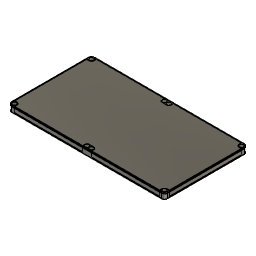
v1.0 (Autodesk Fusion 360 design; units mm, degrees)
Autodesk Fusion 360 part; units mm, degrees
sketch "Sketch1" plane through (0, 0, 0) normal (0, 0, 1) x (1, 0, 0)
  line L0 (192, -6) -> (205, -6) construction
  line L1 (192, -6) -> (179, -6) construction
  circle A0 centre (179, -188) radius 2
  circle A1 centre (13, -188) radius 2
  line L2 (13, -6) -> (13, -16) construction
  circle A2 centre (205, -16) radius 2
  line L3 (13, -198) -> (13, -188) construction
  line L4 (384, -198) -> (371, -198) construction
  line L5 (179, -26) -> (13, -26)
  line L6 (192, -198) -> (179, -198) construction
  line L7 (384, -6) -> (371, -6) construction
  line L8 (179, -6) -> (179, -26) construction
  line L9 (192, -198) -> (0, -198)
  line L10 (205, -198) -> (205, -188) construction
  line L11 (0, -198) -> (0, -6)
  circle A3 centre (179, -16) radius 2
  line L12 (384, -198) -> (384, -6)
  line L13 (371, -26) -> (205, -26)
  line L14 (371, -198) -> (371, -188) construction
  line L15 (205, -26) -> (205, -178)
  line L16 (13, -178) -> (179, -178)
  line L17 (0, -198) -> (13, -198) construction
  line L18 (205, -198) -> (205, -178) construction
  circle A4 centre (205, -188) radius 2
  line L19 (0, -198) -> (13, -198) construction
  line L20 (371, -6) -> (371, -16) construction
  line L21 (192, -6) -> (179, -6) construction
  circle A5 centre (13, -16) radius 2
  circle A6 centre (371, -16) radius 2
  line L22 (192, -6) -> (192, -198) construction
  line L23 (179, -6) -> (179, -16) construction
  line L24 (371, -6) -> (371, -26) construction
  line L25 (205, -6) -> (205, -16) construction
  line L26 (13, -26) -> (13, -178)
  line L27 (384, -6) -> (0, -6)
  line L28 (179, -198) -> (179, -188) construction
  line L29 (13, -198) -> (13, -178) construction
  line L30 (0, -6) -> (13, -6) construction
  line L31 (179, -178) -> (179, -26)
  line L32 (192, -198) -> (205, -198) construction
  line L33 (0, -6) -> (0, -198)
  line L34 (205, -178) -> (371, -178)
  circle A7 centre (371, -188) radius 2
  line L35 (384, -6) -> (371, -6) construction
  line L36 (371, -178) -> (371, -26)
  line L37 (0, -198) -> (384, -198)
  line L38 (192, -198) -> (205, -198) construction
  line L39 (384, -6) -> (384, 12) construction
  line L40 (0, -6) -> (-10.6066, 4.6066) construction
  line L41 (0, -6) -> (15, -6) construction
  circle A8 centre (-5.3033, -0.6967) radius 7.5
  line L42 (0, -198) -> (-10.6066, -208.6066) construction
  line L43 (384, -198) -> (394.6066, -208.6066) construction
  line L44 (384, -198) -> (399, -198) construction
  line L45 (384, -6) -> (394.6066, 4.6066) construction
  line L46 (384, -6) -> (399, -6) construction
  circle A9 centre (389.3033, -0.6967) radius 7.5
  circle A10 centre (389.3033, -203.3033) radius 7.5
  circle A11 centre (-5.3033, -203.3033) radius 7.5
  line L47 (-12.7709, 0) -> (-12.8033, -203.3021)
  line L48 (-5.3033, -210.8033) -> (389.3033, -210.8033)
  line L49 (396.8033, -203.3033) -> (396.8033, -0.6967)
  line L50 (-5.3033, 6.8033) -> (389.3033, 6.8033)
  point P0 (13, -13)
  dimension "d13" = 192
  dimension "d14" = 192
  dimension "d15" = 384
  dimension "d16" = 384
  dimension "d20" = 13
  dimension "d21" = 10
  dimension "d22" = 4
  dimension "d23" = 13
  dimension "d24" = 10
  dimension "d25" = 13
  dimension "d26" = 10
  dimension "d27" = 13
  dimension "d28" = 10
  dimension "d29" = 13
  dimension "d30" = 10
  dimension "d31" = 13
  dimension "d32" = 10
  dimension "d33" = 13
  dimension "d34" = 10
  dimension "d35" = 13
  dimension "d36" = 10
  dimension "d37" = 4
  dimension "d38" = 4
  dimension "d39" = 4
  dimension "d40" = 4
  dimension "d41" = 4
  dimension "d42" = 4
  dimension "d43" = 4
  dimension "d44" = 13
  dimension "d45" = 20
  dimension "d46" = 13
  dimension "d47" = 20
  dimension "d48" = 13
  dimension "d49" = 20
  dimension "d50" = 13
  dimension "d51" = 20
  dimension "d69" = 135
  dimension "d70" = 15
  dimension "d71" = 15
  dimension "d72" = 45
  dimension "d73" = 15
  dimension "d74" = 15
  dimension "d75" = 45
  constraint perpendicular L11 L30
  constraint perpendicular L2 L30
  constraint coincident L2.end A5.centre
  constraint perpendicular L7 L12
  constraint perpendicular L7 L20
  constraint perpendicular L4 L12
  constraint perpendicular L14 L37
  constraint perpendicular L19 L33
  constraint perpendicular L3 L19
  constraint midpoint L0.start L27
  constraint perpendicular L22 L37
  constraint perpendicular L6 L22
  constraint perpendicular L9 L28
  constraint perpendicular L21 L22
  constraint perpendicular L21 L23
  constraint perpendicular L0 L22
  constraint perpendicular L25 L27
  constraint perpendicular L22 L32
  constraint perpendicular L10 L32
  constraint coincident A1.centre L3.end
  constraint coincident A3.centre L23.end
  constraint coincident A0.centre L28.end
  constraint coincident A2.centre L25.end
  constraint coincident L10.end A4.centre
  constraint coincident L14.end A7.centre
  constraint coincident L20.end A6.centre
  constraint perpendicular L11 L17
  constraint perpendicular L17 L29
  constraint perpendicular L1 L22
  constraint perpendicular L1 L8
  constraint horizontal L16
  constraint vertical L31
  constraint horizontal L5
  constraint vertical L26
  constraint perpendicular L22 L38
  constraint perpendicular L18 L38
  constraint perpendicular L20 L35
  constraint perpendicular L24 L35
  constraint horizontal L34
  constraint vertical L36
  constraint horizontal L13
  constraint vertical L15
  constraint perpendicular L7 L39
  constraint horizontal L41
  constraint coincident L40.end A8
  constraint coincident L11.end A8
  constraint horizontal L44
  constraint horizontal L46
  constraint coincident L45.end A9
  constraint coincident L7.start A9
  constraint coincident L43.end A10
  constraint coincident L4.start A10
  constraint coincident L42.end A11
  constraint coincident L9.end A11
  constraint coincident A8 L47.start
  constraint coincident A11 L47.end
  constraint tangent A11 L47
  constraint coincident A11 L48.start
  constraint coincident A10 L48.end
  constraint tangent A10 L48
  constraint coincident A10 L49.start
  constraint coincident A9 L49.end
  constraint tangent A9 L49
  constraint perpendicular L46 L49
  constraint coincident A8 L50.start
  constraint coincident A9 L50.end
  constraint tangent A9 L50
  constraint perpendicular L49 L50
  measures "d13" distance of L11.end L9.end
  measures "d14" distance of L4.start L7.start
  measures "d15" distance of L7.start L11.end
  measures "d16" distance of L4.start L9.end
  measures "d20" distance of L2.start L11.end
  measures "d21" distance of L2.start L2.end
  measures "d22" diameter of A5
  measures "d23" distance of L7.end L7.start
  measures "d24" distance of L7.end L20.end
  measures "d25" distance of L4.end L4.start
  measures "d26" distance of L4.end L14.end
  measures "d27" distance of L3.start L9.end
  measures "d28" distance of L3.start A1.centre
  measures "d29" distance of L6.end L6.start
  measures "d30" distance of L6.end A0.centre
  measures "d31" distance of L0.start L1.end
  measures "d32" distance of A3.centre L1.end
  measures "d33" distance of L0.start L0.end
  measures "d34" distance of A2.centre L0.end
  measures "d35" distance of L10.start L6.start
  measures "d36" distance of L10.end L10.start
  measures "d37" diameter of A1
  measures "d38" diameter of A3
  measures "d39" diameter of A0
  measures "d40" diameter of A2
  measures "d41" diameter of A4
  measures "d42" diameter of A7
  measures "d43" diameter of A6
  measures "d44" distance of L9.end L3.start
  measures "d45" distance of L16.start L3.start
  measures "d46" distance of L0.start L1.end
  measures "d47" distance of L5.start L1.end
  measures "d48" distance of L6.start L10.start
  measures "d49" distance of L10.start L15.end
  measures "d50" distance of L7.start L7.end
  measures "d51" distance of L13.start L7.end
  measures "d69" angle of L40 L41
  measures "d70" distance of L11.end L40.end
  measures "d71" distance of L9.end L42.end
  measures "d72" angle of L43 L44
  measures "d73" distance of L4.start L43.end
  measures "d74" distance of L7.start L45.end
  measures "d75" angle of L45 L46
extrude "Extrude1" add sketch "Sketch1" along normal blind 2 contours L9 L37 A10 A11 L48 | L9 L11 L12 L27 L33 L37 | L11 L33 A8 A11 L47 | A11 | L12 A9 A10 L49 | A10 | L27 A8 A9 L50 | A8 L47 | A9 picked at (-7.7336, 1.0063) makes body 1
sketch "Sketch3" plane through (0, 0, 2) normal (0, 0, 1) x (-1, 0, 0)
  circle A0 centre (-179, 16) radius 2
  circle A1 centre (-205, 188) radius 2
  circle A2 centre (-179, 188) radius 2
  circle A3 centre (-13, 16) radius 2
  circle A4 centre (-205, 16) radius 2
  circle A5 centre (-13, 188) radius 2
  circle A6 centre (-371, 16) radius 2
  line L0 (-179, 26) -> (-179, 178)
  line L1 (-179, 178) -> (-13, 178)
  line L2 (-13, 178) -> (-13, 26)
  line L3 (-13, 26) -> (-179, 26)
  line L4 (-371, 26) -> (-371, 178)
  line L5 (-371, 178) -> (-205, 178)
  line L6 (-205, 178) -> (-205, 26)
  line L7 (-205, 26) -> (-371, 26)
  circle A7 centre (-371, 188) radius 2
  line L8 (12.7709, 0) -> (12.8033, 203.3021)
  arc A8 (12.8033, 203.3021) -> (5.3033, 210.8033) centre (5.3033, 203.3033) ccw
  line L9 (5.3033, 210.8033) -> (-389.3033, 210.8033)
  arc A9 (-389.3033, 210.8033) -> (-396.8033, 203.3033) centre (-389.3033, 203.3033) ccw
  line L10 (-396.8033, 203.3033) -> (-396.8033, 0.6967)
  arc A10 (-396.8033, 0.6967) -> (-389.3033, -6.8033) centre (-389.3033, 0.6967) ccw
  line L11 (-389.3033, -6.8033) -> (5.3033, -6.8033)
  arc A11 (5.3033, -6.8033) -> (12.7709, 0) centre (5.3033, 0.6967) ccw
  circle A12 centre (5.3033, 0.6967) radius 6.5
  circle A13 centre (5.3033, 203.3033) radius 6.5
  circle A14 centre (-389.3033, 203.3033) radius 6.5
  circle A15 centre (-389.3033, 0.6967) radius 6.5
  line L12 (-389.3033, -5.8033) -> (5.3033, -5.8033)
  line L13 (11.8033, 0.6967) -> (11.8033, 203.3033)
  line L14 (5.3033, 209.8033) -> (-389.3033, 209.8033)
  line L15 (-395.8033, 203.3033) -> (-395.8033, 0.6967)
  line L16 (-192, -5.8033) -> (-192, 209.8033) construction
  circle A16 centre (-186, 0.1967) radius 6
  circle A17 centre (-198, 0.1967) radius 6
  circle A18 centre (-186, 203.8033) radius 6
  circle A19 centre (-198, 203.8033) radius 6
  line L17 (-180, 203.8033) -> (-180, 209.8033)
  line L18 (-186, 197.8033) -> (-198, 197.8033)
  line L19 (-204, 203.8033) -> (-204, 209.8033)
  line L20 (-186, 6.1967) -> (-198, 6.1967)
  line L21 (-204, 0.1967) -> (-204, -5.8033)
  line L22 (-180, 0.1967) -> (-180, -5.8033)
  line L23 (-383.662, 197.9997) -> (-384, 6)
  line L24 (0.338, 197.9997) -> (-383.662, 197.9997)
  line L25 (0, 6) -> (0.338, 197.9997)
  line L26 (-384, 6) -> (0, 6)
  line L27 (5.3033, 7.1967) -> (11.8033, 7.1967)
  line L28 (-1.1967, 0.6967) -> (-1.1967, -5.8033)
  line L29 (-382.8033, 0.6967) -> (-382.8033, -5.8033)
  line L30 (-389.3033, 7.1967) -> (-395.8033, 7.1967)
  line L31 (-389.3033, 196.8033) -> (-395.8033, 196.8033)
  line L32 (-382.8033, 203.3033) -> (-382.8033, 209.8033)
  line L33 (5.3033, 196.8033) -> (11.8033, 196.8033)
  line L34 (-1.1967, 203.3033) -> (-1.1967, 209.8033)
  dimension "d76" = 13
  dimension "d77" = 13
  dimension "d78" = 13
  dimension "d79" = 13
  dimension "d80" = 6
  dimension "d81" = 6
  dimension "d82" = 6
  dimension "d83" = 6
  dimension "d84" = 192
  dimension "d85" = 192
  dimension "d86" = 384
  dimension "d87" = 384
  constraint concentric A11 A12
  constraint concentric A8 A13
  constraint concentric A9 A14
  constraint concentric A10 A15
  constraint coincident A15 L12.start
  constraint coincident A12 L12.end
  constraint tangent A12 L12
  constraint parallel L11 L12
  constraint coincident A12 L13.start
  constraint coincident A13 L13.end
  constraint tangent A13 L13
  constraint coincident A13 L14.start
  constraint coincident A14 L14.end
  constraint tangent A14 L14
  constraint coincident A14 L15.start
  constraint coincident A15 L15.end
  constraint tangent A15 L15
  constraint parallel L10 L15
  constraint midpoint L12 L16.start
  constraint midpoint L14 L16.end
  constraint tangent L12 A16
  constraint tangent L16 A16
  constraint tangent L16 A17
  constraint tangent L12 A17
  constraint tangent L16 A18
  constraint tangent L14 A18
  constraint tangent L16 A19
  constraint tangent L14 A19
  constraint coincident A18 L17.start
  constraint coincident L14 L17.end
  constraint tangent A18 L17
  constraint vertical L17
  constraint coincident A18 L18.start
  constraint coincident A19 L18.end
  constraint tangent A19 L18
  constraint coincident A19 L19.start
  constraint coincident L14 L19.end
  constraint tangent A19 L19
  constraint coincident A16 L20.start
  constraint coincident A17 L20.end
  constraint tangent A17 L20
  constraint horizontal L20
  constraint coincident A17 L21.start
  constraint coincident L12 L21.end
  constraint tangent A17 L21
  constraint perpendicular L12 L21
  constraint coincident A16 L22.start
  constraint coincident L12 L22.end
  constraint tangent A16 L22
  constraint perpendicular L12 L22
  constraint coincident A12 L27.start
  constraint coincident L13 L27.end
  constraint tangent A12 L27
  constraint horizontal L27
  constraint coincident A12 L28.start
  constraint coincident L12 L28.end
  constraint tangent A12 L28
  constraint perpendicular L12 L28
  constraint coincident A15 L29.start
  constraint coincident L12 L29.end
  constraint tangent A15 L29
  constraint perpendicular L12 L29
  constraint coincident A15 L30.start
  constraint coincident L15 L30.end
  constraint tangent A15 L30
  constraint perpendicular L15 L30
  constraint coincident A14 L31.start
  constraint coincident L15 L31.end
  constraint tangent A14 L31
  constraint perpendicular L15 L31
  constraint coincident A14 L32.start
  constraint coincident L14 L32.end
  constraint tangent A14 L32
  constraint vertical L32
  constraint coincident A13 L33.start
  constraint coincident L13 L33.end
  constraint tangent A13 L33
  constraint horizontal L33
  constraint coincident A13 L34.start
  constraint coincident L14 L34.end
  constraint tangent A13 L34
  constraint vertical L34
  measures "d76" diameter of A12
  measures "d77" diameter of A13
  measures "d78" diameter of A14
  measures "d79" diameter of A15
  measures "d80" radius of A16
  measures "d81" radius of A17
  measures "d82" radius of A18
  measures "d83" radius of A19
  measures "d84" distance of L23.start L23.end
  measures "d85" distance of L25.start L24.start
  measures "d86" distance of L23.start L24.start
  measures "d87" distance of L25.start L23.end
extrude "Extrude3" add sketch "Sketch3" along normal blind 10.5 contours L8 A8 L9 A9 L10 A10 L11 A11 | A12 | A12 L13 L27 | A12 L12 L28 | A13 L13 L33 | L12 A16 L22 | A13 | L12 A16 A17 | A16 L26 | A13 L14 L34 | L12 A17 L21 | A17 L26 | A16 A17 L26 | L14 A18 L17 | A15 L12 L29 | L14 A18 A19 | A18 L24 | A15 | L14 A19 L19 | A19 L24 | A18 A19 L24 | A15 L15 L30 | A14 L14 L32 | A14 L15 L31 | A14 picked at (-184.1807, -0.0522) picked at (-196.552, 2.8723) picked at (-187.7318, 201.8336) picked at (-197.7109, 205.5309) bodies 1
sketch "Sketch4" plane through (0, 0, 12.5) normal (0, 0, 1) x (-1, 0, 0)
  arc A0 (-199.5237, 6) -> (-204, 0.1967) centre (-198, 0.1967) ccw
  line L0 (-204, 0.1967) -> (-204, -5.8033)
  line L1 (-204, -5.8033) -> (-382.8033, -5.8033)
  arc A1 (-382.8033, 0.6967) -> (-389.3033, 7.1967) centre (-389.3033, 0.6967) ccw
  line L2 (-395.8033, 7.1967) -> (-395.8033, 196.8033)
  arc A2 (-389.3033, 196.8033) -> (-382.8033, 203.3033) centre (-389.3033, 203.3033) ccw
  line L3 (-382.8033, 209.8033) -> (-204, 209.8033)
  line L4 (-204, 209.8033) -> (-204, 203.8033)
  arc A3 (-204, 203.8033) -> (-199.5226, 197.9997) centre (-198, 203.8033) ccw
  line L5 (-199.5226, 197.9997) -> (-184.4774, 197.9997)
  arc A4 (-184.4774, 197.9997) -> (-180, 203.8033) centre (-186, 203.8033) ccw
  line L6 (-180, 203.8033) -> (-180, 209.8033)
  line L7 (-180, 209.8033) -> (-1.1967, 209.8033)
  arc A5 (-1.1967, 203.3033) -> (5.3033, 196.8033) centre (5.3033, 203.3033) ccw
  line L8 (11.8033, 196.8033) -> (11.8033, 7.1967)
  arc A6 (5.3033, 7.1967) -> (-1.1967, 0.6967) centre (5.3033, 0.6967) ccw
  line L9 (-1.1967, -5.8033) -> (-180, -5.8033)
  line L10 (-180, -5.8033) -> (-180, 0.1967)
  arc A7 (-180, 0.1967) -> (-184.4763, 6) centre (-186, 0.1967) ccw
  line L11 (-184.4763, 6) -> (-199.5237, 6)
  arc A8 (5.3033, -6.8033) -> (12.7709, 0) centre (5.3033, 0.6967) ccw
  line L12 (12.7709, 0) -> (12.8033, 203.3021)
  arc A9 (12.8033, 203.3021) -> (5.3033, 210.8033) centre (5.3033, 203.3033) ccw
  line L13 (5.3033, 210.8033) -> (-389.3033, 210.8033)
  arc A10 (-389.3033, 210.8033) -> (-396.8033, 203.3033) centre (-389.3033, 203.3033) ccw
  line L14 (-396.8033, 203.3033) -> (-396.8033, 0.6967)
  arc A11 (-396.8033, 0.6967) -> (-389.3033, -6.8033) centre (-389.3033, 0.6967) ccw
  line L15 (-389.3033, -6.8033) -> (5.3033, -6.8033)
  circle A12 centre (5.3033, 0.6967) radius 5.1
  circle A13 centre (-186, 0.1967) radius 5.1
  circle A14 centre (-198, 0.1967) radius 5.1
  circle A15 centre (-389.3033, 0.6967) radius 5.1
  circle A16 centre (-389.3033, 203.3033) radius 5.1
  circle A17 centre (-198, 203.8033) radius 5.1
  circle A18 centre (-186, 203.8033) radius 5.1
  circle A19 centre (5.3033, 203.3033) radius 5.1
  line L16 (5.3033, 196.8033) -> (11.8033, 196.8033)
  line L17 (11.8033, 7.1967) -> (5.3033, 7.1967)
  line L18 (-1.1967, 0.6967) -> (-1.1967, -5.8033)
  line L19 (-382.8033, -5.8033) -> (-382.8033, 0.6967)
  line L20 (-389.3033, 7.1967) -> (-395.8033, 7.1967)
  line L21 (-395.8033, 196.8033) -> (-389.3033, 196.8033)
  line L22 (-382.8033, 203.3033) -> (-382.8033, 209.8033)
  line L23 (-1.1967, 209.8033) -> (-1.1967, 203.3033)
  dimension "d90" = 10.2
  dimension "d91" = 10.2
  dimension "d92" = 10.2
  dimension "d93" = 10.2
  dimension "d94" = 10.2
  dimension "d95" = 10.2
  dimension "d96" = 10.2
  dimension "d97" = 10.2
  constraint concentric A6 A12
  constraint concentric A7 A13
  constraint concentric A0 A14
  constraint concentric A1 A15
  constraint concentric A2 A16
  constraint concentric A3 A17
  constraint concentric A4 A18
  constraint concentric A5 A19
  measures "d90" diameter of A12
  measures "d91" diameter of A13
  measures "d92" diameter of A14
  measures "d93" diameter of A15
  measures "d94" diameter of A16
  measures "d95" diameter of A17
  measures "d96" diameter of A18
  measures "d97" diameter of A19
extrude "Extrude4" cut sketch "Sketch4" against normal blind 3.2 contours A12 | A13 | A14 | A15 | A16 | A17 | A18 | A19 bodies 1
extrude "Extrude5" add 1 faces at (386.3311, -209.467, 12.5) along direction (0, 0, 1) blind 3 separate body on bodies 1 makes body 2
sketch "Sketch5" plane through (0, 0, 15.5) normal (0, 0, 1) x (-1, 0, 0)
  circle A0 centre (-198, 203.8033) radius 5.1
  circle A1 centre (-186, 0.1967) radius 5.1
  circle A2 centre (-198, 0.1967) radius 5.1
  circle A3 centre (-186, 203.8033) radius 5.1
  circle A4 centre (-389.3033, 203.3033) radius 5.1
  circle A5 centre (5.3033, 0.6967) radius 5.1
  circle A6 centre (-389.3033, 0.6967) radius 5.1
  circle A7 centre (5.3033, 203.3033) radius 5.1
  arc A8 (-1.1967, 203.3033) -> (5.3033, 196.8033) centre (5.3033, 203.3033) ccw
  line L0 (5.3033, 196.8033) -> (11.8033, 196.8033)
  line L1 (11.8033, 196.8033) -> (11.8033, 7.1967)
  line L2 (11.8033, 7.1967) -> (5.3033, 7.1967)
  arc A9 (5.3033, 7.1967) -> (-1.1967, 0.6967) centre (5.3033, 0.6967) ccw
  line L3 (-1.1967, 0.6967) -> (-1.1967, -5.8033)
  line L4 (-1.1967, -5.8033) -> (-180, -5.8033)
  line L5 (-180, -5.8033) -> (-180, 0.1967)
  arc A10 (-180, 0.1967) -> (-184.4763, 6) centre (-186, 0.1967) ccw
  line L6 (-184.4763, 6) -> (-199.5237, 6)
  arc A11 (-199.5237, 6) -> (-204, 0.1967) centre (-198, 0.1967) ccw
  line L7 (-204, 0.1967) -> (-204, -5.8033)
  line L8 (-204, -5.8033) -> (-382.8033, -5.8033)
  line L9 (-382.8033, -5.8033) -> (-382.8033, 0.6967)
  arc A12 (-382.8033, 0.6967) -> (-389.3033, 7.1967) centre (-389.3033, 0.6967) ccw
  line L10 (-389.3033, 7.1967) -> (-395.8033, 7.1967)
  line L11 (-395.8033, 7.1967) -> (-395.8033, 196.8033)
  line L12 (-395.8033, 196.8033) -> (-389.3033, 196.8033)
  arc A13 (-389.3033, 196.8033) -> (-382.8033, 203.3033) centre (-389.3033, 203.3033) ccw
  line L13 (-382.8033, 203.3033) -> (-382.8033, 209.8033)
  line L14 (-382.8033, 209.8033) -> (-204, 209.8033)
  line L15 (-204, 209.8033) -> (-204, 203.8033)
  arc A14 (-204, 203.8033) -> (-199.5226, 197.9997) centre (-198, 203.8033) ccw
  line L16 (-199.5226, 197.9997) -> (-184.4774, 197.9997)
  arc A15 (-184.4774, 197.9997) -> (-180, 203.8033) centre (-186, 203.8033) ccw
  line L17 (-180, 203.8033) -> (-180, 209.8033)
  line L18 (-180, 209.8033) -> (-1.1967, 209.8033)
  line L19 (-1.1967, 209.8033) -> (-1.1967, 203.3033)
  arc A16 (5.3033, -6.8033) -> (12.7709, 0) centre (5.3033, 0.6967) ccw
  line L20 (12.7709, 0) -> (12.8033, 203.3021)
  arc A17 (12.8033, 203.3021) -> (5.3033, 210.8033) centre (5.3033, 203.3033) ccw
  line L21 (5.3033, 210.8033) -> (-389.3033, 210.8033)
  arc A18 (-389.3033, 210.8033) -> (-396.8033, 203.3033) centre (-389.3033, 203.3033) ccw
  line L22 (-396.8033, 203.3033) -> (-396.8033, 0.6967)
  arc A19 (-396.8033, 0.6967) -> (-389.3033, -6.8033) centre (-389.3033, 0.6967) ccw
  line L23 (-389.3033, -6.8033) -> (5.3033, -6.8033)
  circle A20 centre (5.3033, 0.6967) radius 7.5
  circle A21 centre (-389.3033, 0.6967) radius 7.5
  circle A22 centre (-389.3033, 203.3033) radius 7.5
  circle A23 centre (5.3033, 203.3033) radius 7.5
  line L24 (12.8033, 203.3021) -> (12.7709, 0)
  line L25 (5.3033, -6.8033) -> (-389.3033, -6.8033)
  line L26 (-396.8033, 0.6967) -> (-396.8033, 203.3033)
  line L27 (-389.3033, 210.8033) -> (5.3033, 210.8033)
  constraint concentric A5 A20
  constraint concentric A6 A21
  constraint concentric A4 A22
  constraint concentric A7 A23
  constraint coincident L20.end A17.start
  constraint coincident A16.end L20.start
  constraint coincident A16.start L23.end
  constraint coincident A19.end L23.start
  constraint tangent A21 L25
  constraint coincident L22.end A19.start
  constraint coincident A18.end L22.start
  constraint tangent A22 L26
  constraint coincident L21.end A18.start
  constraint coincident A17.end L21.start
extrude "Extrude6" add sketch "Sketch5" along normal blind 0.5 contours A0 | A1 | A2 | A3 | A4 | A5 | A6 | A7 | A8 L0 L19 A17 A23 | A8 L0 L19 A23 | L0 L1 L2 L3 L4 L5 A10 L6 A11 L7 L8 L9 L10 L11 L12 L13 L14 L15 A14 L16 A15 L17 L18 L19 A20 A21 A22 A23 | L13 L14 L15 A14 L16 A15 L17 L18 L19 L21 A22 A23 L27 | L0 L1 L2 L20 A20 A23 L24 | L12 A13 L13 A18 A22 | L2 A9 L3 A16 L20 A20 L24 | L10 L11 L12 L22 A21 A22 L26 | L12 A13 L13 A22 | L2 A9 L3 A20 | L9 A12 L10 A19 A21 | L3 L4 L5 A10 L6 A11 L7 L8 L9 L23 A20 A21 L25 | L9 A12 L10 A21 bodies 2
equation "d16 = ( 192 * 2 ) * 1 mm"
equation "d87 = ( 192 * 2 ) * 1 mm"
